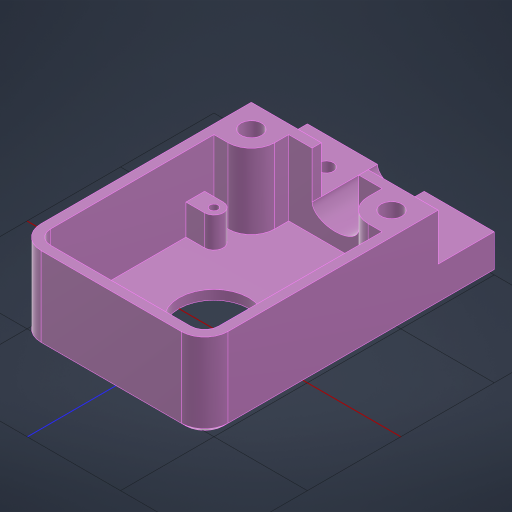
# Autodesk Inventor part: LED-Ring_Camera-Housing
Saved by Autodesk Inventor 2023.2 (Build 272271030, 271C)
## iProperties
Created: 2023-02-19
Part Number: LED-Ring_Camera-Housing
Material: Generisch
Document SubType Name: Modeling
Designer: Stefan
Mass: 14.1491 g
Surface Area: 110.678 cm^2
Volume: 14.1491 cm^3
Density: 1 g/cm^3
Appearance: Glatt - Violett
Author: Stefan
Autodesk Inventor part; units mm, degrees
ref_plane "YZ Plane" through (0, 0, 0) normal (1, 0, 0) x (0, 1, 0)
ref_plane "XZ Plane" through (0, 0, 0) normal (0, 1, 0) x (-1, 0, 0)
ref_plane "XY Plane" through (0, 0, 0) normal (0, 0, 1) x (1, 0, 0)
sketch "Skizze1" plane through (0, 0, 0) normal (0, 1, 0) x (-1, 0, 0)
  arc A0 (20, 17) -> (15, 22) centre (15, 17) ccw
  arc A1 (-15, 22) -> (-20, 17) centre (-15, 17) ccw
  line L0 (14, -12) -> (18, -12)
  arc A2 (14, -12) -> (14, -16) centre (14, -14) ccw
  line L1 (18, -16) -> (14, -16)
  line L2 (-14, -16) -> (-18, -16)
  arc A3 (-14, -16) -> (-14, -12) centre (-14, -14) ccw
  line L3 (-18, -12) -> (-14, -12)
  line L4 (-14, 12) -> (-18, 12)
  arc A4 (-14, 12) -> (-14, 16) centre (-14, 14) ccw
  line L5 (-18, 16) -> (-14, 16)
  line L6 (14, 16) -> (18, 16)
  arc A5 (14, 16) -> (14, 12) centre (14, 14) ccw
  line L7 (18, 12) -> (14, 12)
  line L8 (14, 14) -> (-14, 14) construction
  line L9 (-14, 14) -> (-14, -14) construction
  line L10 (-14, -14) -> (14, -14) construction
  line L11 (14, -14) -> (14, 14) construction
  line L12 (14, 14) -> (-14, -14) construction
  line L13 (-14, 14) -> (14, -14) construction
  circle A6 centre (0, 0) radius 7.5
  line L14 (20, -40) -> (-20, -40) construction
  line L15 (-20, -40) -> (-20, 22) construction
  line L16 (-20, 22) -> (20, 22) construction
  line L17 (20, 22) -> (20, -40) construction
  line L18 (20, -40) -> (-20, -40)
  line L19 (15, 22) -> (-15, 22)
  line L20 (20, -40) -> (20, 17)
  line L21 (-20, 17) -> (-20, -40)
  line L22 (0, -40) -> (0, 22) construction
  arc A7 (18, 17) -> (15, 20) centre (15, 17) ccw
  arc A8 (-15, 20) -> (-18, 17) centre (-15, 17) ccw
  line L23 (-15, 20) -> (15, 20)
  circle A9 centre (14, 14) radius 0.9
  circle A10 centre (-14, 14) radius 0.9
  circle A11 centre (-14, -14) radius 0.9
  circle A12 centre (14, -14) radius 0.9
  line L24 (20, -28) -> (-20, -28)
  circle A13 centre (-15, -23) radius 5 construction
  circle A14 centre (15, -23) radius 5 construction
  line L25 (-18, -18) -> (-15, -18)
  line L26 (-10, -23) -> (-10, -26)
  line L27 (15, -18) -> (18, -18)
  line L28 (10, -23) -> (10, -26)
  arc A15 (-10, -23) -> (-15, -18) centre (-15, -23) ccw
  arc A16 (15, -18) -> (10, -23) centre (15, -23) ccw
  circle A17 centre (-15, -23) radius 2.25
  circle A18 centre (15, -23) radius 2.25
  line L29 (-18, -18) -> (-18, 17)
  line L30 (18, 17) -> (18, -18)
  line L31 (-10, -26) -> (10, -26)
  point P0 (0, 0)
  point P1 (0, 20)
  point P2 (0, -26)
  point P3 (-15, -18)
  point P4 (-12, -14)
  point P5 (-12, -19)
  point P6 (12, -14)
  point P7 (12, -19)
  dimension "d2" = 15
  dimension "d3" = 40
  dimension "d5" = 22
  dimension "d7" = 5
  dimension "d10" = 2
  dimension "d14" = 1.8
  dimension "d41" = 12
  dimension "d42" = 2
  dimension "d43" = 2
  dimension "d45" = 4.5
  dimension "d49" = 10
  dimension "d50" = 28
  dimension "d51" = 2
  dimension "d52" = 28
  constraints: 64 end point, 29 point on circle, 22 tangent, 19 centre point, 15 perpendicular, 15 point on line, 12 coincident, 11 equal radius, 6 parallel, 4 collinear, 4 midpoint, 3 horizontal, 1 other
  measures "d2" diameter of A6
  measures "d3" distance between parallel lines of L15 L17
  measures "d5" distance from line of L16 point (0, 0)
  measures "d7" radius of A0
  measures "d10" radius of A5
  measures "d14" diameter of A9
  measures "d41" distance between parallel lines of L14 L24
  measures "d42" radial gap between concentric circles of A8 A1
  measures "d43" radial gap between concentric circles of A7 A0
  measures "d45" diameter of A17
  measures "d49" diameter of A13
  measures "d50" distance from line of L24 point (0, 0)
  measures "d51" distance between parallel lines of L24 L31
  measures "d52" distance of L8.start L8.end
extrude "Extrusion1" add sketch "Skizze1" against normal blind 2 contours L20 L24 L21 A1 L19 A0 | L20 L18 L21 L24 | A2 L1 L30 L27 A16 L28 L31 L26 A15 L25 L29 L2 A3 L3 L4 A4 L5 A8 L23 A7 L6 A5 L7 L0 | L0 L30 L1 A2 | L7 A5 L6 L30 | L5 A4 L4 L29 | L3 A3 L2 L29 | A9 | A10 | A11 | A12 | A17 | A18
extrude "Extrusion2" add sketch "Skizze1" along normal blind 16 contours L20 L24 L21 A1 L19 A0
extrude "Extrusion3" add sketch "Skizze1" along normal blind 6 contours L20 L18 L21 L24
extrude "Extrusion4" add sketch "Skizze1" along normal blind 6.5 contours L0 L30 L1 A2 | L7 A5 L6 L30 | L5 A4 L4 L29 | L3 A3 L2 L29
sketch "Skizze2" plane through (0, -2, 0) normal (0, -1, 0) x (1, 0, 0)
  arc A0 (-15, 22) -> (-20, 17) centre (-15, 17) ccw projected
  line L0 (-20, 17) -> (-20, -40) projected
  line L1 (-20, -40) -> (20, -40) projected
  line L2 (20, -40) -> (20, 17) projected
  arc A1 (20, 17) -> (15, 22) centre (15, 17) ccw projected
  line L3 (15, 22) -> (-15, 22) projected
  circle A2 centre (0, 0) radius 7.5 projected
  line L4 (15, 22) -> (-15, 22) projected
  line L5 (0, 22) -> (0, -40) construction
  point P0 (10, -34)
  point P1 (-10, -34)
  dimension "d25" = 20
  dimension "d26" = 6
  constraints: 2 end point, 2 midpoint, 1 symmetric about line
  measures "d25" distance of point (-10, -34) point (10, -34)
  measures "d26" distance from line of L1 point (10, -34)
hole "Bohrung1" at (10, -2, -34) at (-10, -2, -34) direction (0, 1, 0) diameter 3.2 end through all counterbore diameter 6.5 counterbore depth 3.4 clearance for "Inbusschraube DIN EN ISO 4762" size "M3" standard "DIN"
sketch "Skizze3" plane through (20, -2, -40) normal (0, 0, -1) x (-1, 0, 0)
  line L0 (0, 8) -> (40, 8) projected
  line L1 (40, 8) -> (40, 18) projected
  line L2 (0, 18) -> (40, 18) projected
  line L3 (0, 8) -> (0, 18) projected
  line L4 (0, 0) -> (0, 8) projected
  line L5 (40, 0) -> (0, 0) projected
  line L6 (40, 0) -> (40, 8) projected
  line L7 (0, 8) -> (40, 8) projected
  line L8 (0, 8) -> (40, 8) projected
  ellipse E0 centre (20, 8) end of major axis (25, 8) minor radius 3
  line L9 (0, 8) -> (40, 8) projected
  line L10 (15, 8) -> (15, 18)
  line L11 (5, 18) -> (35, 18) projected
  line L12 (15, 18) -> (25, 18)
  line L13 (25, 8) -> (25, 18)
  point P0 (20, 2)
  dimension "d37" = 3
  dimension "d38" = 5
  constraints: 6 end point, 5 point on line, 2 perpendicular, 1 midpoint, 1 vertical, 4 other
extrude "Extrusion5" cut sketch "Skizze3" against normal up to surface (14 mm away) contours E0 L0 | L10 L2 L13 E0 | L0 E0
extrude "Extrusion6" add sketch "Skizze1" along normal blind 10 contours A17 | A18
chamfer "Fase1" distance 1 angle 45 5 edges at (20, -2, -11.5) (18.5355, -2, 20.5355) (0, -2, 22) (-18.5355, -2, 20.5355) (-20, -2, -11.5)
equation "\"d42\" = d51"
equation "\"d43\" = d51"
